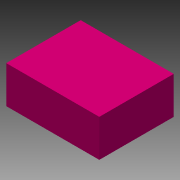
# Autodesk Inventor part: Main board
Saved by Autodesk Inventor 2015 (Build 190159000, 159)
## iProperties
Created: 2015-05-22
Part Number: Main board
Material: 一般
Document SubType Name: Modeling
Designer: kenta
Density: 0.03125 g/cm^3
Appearance: 既定
Mass: 10 g
Surface Area: 304 cm^2
Volume: 320 cm^3
Author: kenta
Autodesk Inventor part; units mm, degrees
ref_plane "YZ Plane" through (0, 0, 0) normal (1, 0, 0) x (0, 1, 0)
ref_plane "XZ Plane" through (0, 0, 0) normal (0, 1, 0) x (-1, 0, 0)
ref_plane "XY Plane" through (0, 0, 0) normal (0, 0, 1) x (1, 0, 0)
sketch "スケッチ1" plane through (0, 0, 0) normal (0, 0, 1) x (1, 0, 0)
  line L0 (-50, 40) -> (50, 40)
  line L1 (50, 40) -> (50, -40)
  line L2 (50, -40) -> (-50, -40)
  line L3 (-50, -40) -> (-50, 40)
  line L4 (-50, 40) -> (50, -40) construction
  line L5 (50, 40) -> (-50, -40) construction
  point P0 (0, 0)
  dimension "d0" = 100
  dimension "d1" = 80
  constraints: 12 end point, 2 midpoint, 2 parallel, 1 horizontal, 1 perpendicular
  measures "d0" distance between parallel lines of L1 L3
  measures "d1" distance of L0.end L1.end
extrude "押し出し1" add sketch "スケッチ1" along normal blind 40
